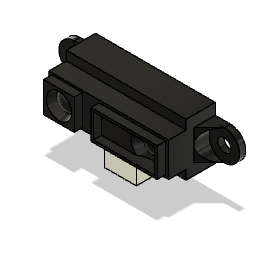
ApoioSensorIR v8 (Autodesk Fusion 360 archive; units mm, degrees)
design "GP2Y0A41SK0F"
Autodesk Fusion 360 part; units mm, degrees
sketch "Base" plane through (0, 0, 0) normal (0, 0, 1) x (1, 0, 0)
  line L0 (-14.75, 6.5) -> (14.75, 6.5)
  line L1 (14.75, 6.5) -> (14.75, -6.5)
  line L2 (14.75, -6.5) -> (-14.75, -6.5)
  line L3 (-14.75, -6.5) -> (-14.75, 6.5)
  line L4 (-18.5, 0) -> (18.5, 0) construction
  circle A0 centre (18.5, 0) radius 1.6
  circle A1 centre (18.5, 0) radius 3.75
  circle A2 centre (-18.5, 0) radius 1.6
  circle A3 centre (-18.5, 0) radius 3.75
  line L5 (-14.75, 3.75) -> (-18.5, 3.75)
  line L6 (14.75, 3.75) -> (18.5, 3.75)
  line L7 (-14.75, -3.75) -> (-18.5, -3.75)
  line L8 (14.75, -3.75) -> (18.5, -3.75)
  line L9 (-6.5, -3.75) -> (-14, -3.75)
  line L10 (-14, -3.75) -> (-14, 3.75)
  line L11 (-14, 3.75) -> (-6.5, 3.75)
  line L12 (-6.5, 3.75) -> (-6.5, -3.75)
  line L13 (-14.75, 4.2) -> (14.75, 4.2)
  line L14 (14.75, -4.2) -> (-14.75, -4.2)
  line L15 (-2.35, 3.6) -> (13.95, 3.6)
  line L16 (13.95, 3.6) -> (13.95, -3.6)
  line L17 (13.95, -3.6) -> (-2.35, -3.6)
  line L18 (-2.35, -3.6) -> (-2.35, 3.6)
  line L19 (-2.35, -3.6) -> (13.95, 3.6) construction
  line L20 (-14, -3.75) -> (-6.5, 3.75) construction
  line L21 (-14.75, -6.5) -> (14.75, 6.5) construction
  line L22 (13.35, -3) -> (-1.75, -3)
  line L23 (-1.75, -3) -> (-1.75, 3)
  line L24 (-1.75, 3) -> (13.35, 3)
  line L25 (13.35, 3) -> (13.35, -3)
  line L26 (0, 0) -> (0, -6.5) construction
  line L27 (-5.05, -6.5) -> (-5.05, -4.2)
  line L28 (5.05, -6.5) -> (5.05, -4.2)
  point P0 (-10.25, 0)
  point P1 (9.45, 0)
  point P2 (-10.25, 0)
  point P3 (5.8, 0)
  dimension "d1" = 29.5
  dimension "d2" = 13
  dimension "d3" = 37
  dimension "d4" = 3.2
  dimension "d5" = 7.5
  dimension "d6" = 19.7
  dimension "d7" = 4.5
  dimension "d8" = 7.5
  dimension "d9" = 7.5
  dimension "d10" = 8.4
  dimension "d11" = 4.2
  dimension "d12" = 16.3
  dimension "d13" = 7.2
  dimension "d14" = 4.15
  dimension "d16" = 0.6
  dimension "d62" = 10.1
  dimension "d63" = 5.05
  constraint horizontal L0
  constraint perpendicular L0 L1
  constraint parallel L0 L2
  constraint parallel L1 L3
  constraint coincident L26.start origin
  constraint perpendicular L1 L4
  constraint midpoint L26.start L4
  constraint coincident L4.end A0.centre
  constraint concentric A0 A1
  constraint coincident L4.start A2.centre
  constraint concentric A2 A3
  constraint equal A0 A2
  constraint equal A1 A3
  constraint coincident L3 L5.start
  constraint coincident A3 L5.end
  constraint parallel L0 L5
  constraint coincident L1 L6.start
  constraint coincident A1 L6.end
  constraint tangent A1 L6
  constraint parallel L0 L6
  constraint tangent A3 L5
  constraint coincident L3 L7.start
  constraint coincident A3 L7.end
  constraint tangent A3 L7
  constraint parallel L2 L7
  constraint coincident L1 L8.start
  constraint coincident A1 L8.end
  constraint tangent A1 L8
  constraint parallel L2 L8
  constraint coincident L4 P2
  constraint coincident L4 P1
  constraint horizontal L9
  constraint perpendicular L9 L10
  constraint parallel L9 L11
  constraint parallel L10 L12
  constraint coincident P2 P0
  constraint coincident L3 L13.start
  constraint coincident L1 L13.end
  constraint perpendicular L1 L13
  constraint coincident L1 L14.start
  constraint coincident L3 L14.end
  constraint perpendicular L3 L14
  constraint horizontal L15
  constraint perpendicular L15 L16
  constraint parallel L15 L17
  constraint parallel L16 L18
  constraint coincident L4 P3
  constraint midpoint P2 L20
  constraint midpoint P3 L19
  constraint midpoint L2 L26.end
  constraint perpendicular L2 L26
  constraint coincident L2 L27.start
  constraint coincident L14 L27.end
  constraint perpendicular L14 L27
  constraint coincident L2 L28.start
  constraint coincident L14 L28.end
  constraint perpendicular L14 L28
  measures "d1" distance of L1.end L2.end
  measures "d2" distance of L0.end L1.end
  measures "d3" distance of L4.start L4.end
  measures "d4" diameter of A0
  measures "d5" diameter of A1
  measures "d6" distance of P2 P1
  measures "d7" distance of L3 P2
  measures "d8" distance of L10.end L11.end
  measures "d9" distance of L9.end L10.end
  measures "d10" distance of L13 L14
  measures "d11" distance of L26.start L14
  measures "d12" distance of L16.end L17.end
  measures "d13" distance of L15.end L16.end
  measures "d14" distance of L12 L18
  measures "d62" distance of L27 L28
  measures "d63" distance of L26 L27
extrude "Extrude1" add sketch "Base" along normal blind 13.5 contours L9 L10 L11 L12 | L15 L16 L17 L18 makes body 1 at (-9, -3.75, 4.5) makes body 2 at (3.0833, 3.6, 4.5)
extrude "Extrude2" add sketch "Base" along normal blind 11.5 contours L1 L3 L13 L14 | L22 L23 L24 L25 bodies 1 2
extrude "Extrude3" add sketch "Base" along normal blind 7.2 contours L0 L1 L3 L13 | L2 L3 L14 L27 | L1 L2 L14 L28 bodies 1
extrude "Extrude10" add sketch "Base" along normal blind 3.3 contours L2 L14 L27 L28 bodies 1
sketch "Fixation" plane through (0, -6.5, 0) normal (0, -1, 0) x (1, 0, 0)
  line L0 (-14.75, 0) -> (14.75, 0)
  line L1 (14.75, 0) -> (14.75, 7.2)
  line L2 (14.75, 7.2) -> (5.05, 7.2)
  line L3 (-14.75, 7.2) -> (-14.75, 0)
  line L4 (14.75, 0) -> (18.5, 0)
  line L5 (14.75, 0) -> (14.75, 5.25)
  line L6 (18.5, 0) -> (18.5, 1.5)
  line L7 (14.75, 5.25) -> (18.5, 1.5)
  line L8 (0, 0) -> (0, 3) construction
  line L9 (-14.75, 5.25) -> (-18.5, 1.5)
  line L10 (-18.5, 0) -> (-18.5, 1.5)
  line L11 (-14.75, 0) -> (-18.5, 0)
  line L12 (-14.75, 0) -> (-14.75, 5.25)
  line L13 (5.05, 7.2) -> (5.05, 3.3)
  line L14 (-5.05, 3.3) -> (-5.05, 7.2)
  line L15 (5.05, 3.3) -> (-5.05, 3.3)
  line L16 (-5.05, 7.2) -> (-14.75, 7.2)
  dimension "d25" = 3.75
  dimension "d26" = 5.25
  dimension "d27" = 1.5
  constraint coincident L0.end L1.start
  constraint perpendicular L1 L4
  constraint perpendicular L0 L5
  constraint perpendicular L4 L6
  constraint coincident L8.start origin
  constraint perpendicular L0 L8
  constraint symmetric L0.end L8 L0.start
  constraint symmetric L4.end L8 L10.start
  constraint symmetric L5.end L8 L9.start
  constraint symmetric L6.end L8 L9.end
  measures "d25" distance of L0.end L4.end
  measures "d26" distance of L0.end L5.end
  measures "d27" distance of L4.end L6.end
extrude "Extrude5" add sketch "Fixation" along normal mid plane 7.5 from surface at -6.5 contours L3 L9 L10 L11 L12 | L1 L4 L5 L6 L7 bodies 1
extrude "Extrude6" cut sketch "Base" along normal through all contours A3 | A1 | A0 | A2 bodies 1
extrude "Extrude7" add sketch "Base" along normal blind 1.5 contours A3 | A1 bodies 1
ref_plane "WorkPlane2" through (5.8, 0, 10) normal (0, 0, 1) x (1, 0, 0)
sketch "Detector_Fitting1" plane through (0, 0, 11.5) normal (0, 0, 1) x (1, 0, 0)
  line L0 (13.35, 3) -> (-1.75, 3)
  line L1 (-1.75, 3) -> (-1.75, -3)
  line L2 (-1.75, -3) -> (13.35, -3)
  line L3 (13.35, -3) -> (13.35, 3)
  line L4 (0, 0) -> (9.45, 0) construction
  circle A0 centre (9.45, 0) radius 4
  dimension "d34" = 9.45
  dimension "d35" = 8
  constraint coincident L4.start origin
  constraint parallel L0 L4
  constraint coincident L4.end A0.centre
  measures "d34" distance of L4.start L4.end
  measures "d35" diameter of A0
sketch "Detector_Fitting2" plane through (5.8, 0, 10) normal (0, 0, 1) x (1, 0, 0)
  line L0 (0, 0) -> (3.625, 0)
  circle A0 centre (3.625, 0) radius 2.375
  dimension "d38" = 3.625
  dimension "d39" = 4.75
  constraint coincident L0.start origin
  constraint horizontal L0
  constraint coincident L0.end A0.centre
  measures "d38" distance of L0.start L0.end
  measures "d39" diameter of A0
loft "Loft1" cut profiles "Detector_Fitting1", "Detector_Fitting2" section 1 contours L0 L2 L3 A0 | L0 A0 | L3 A0 | L2 A0 section 2 bodies 1
extrude "Extrude8" add 1 faces at (-1.6833, -4.2, 10.0667) along direction (0, 1, 0) up to surface (1.2 mm away) on bodies 1 bodies 1
extrude "Extrude9" add 1 faces at (4.9167, 4.2, 10.0667) along direction (0, -1, 0) up to surface (1.2 mm away) on bodies 1 bodies 1
ref_plane "WorkPlane4" through (-10.25, 0, 11.5) normal (0, 0, 1) x (1, 0, 0)
sketch "Emitter_Fitting1" plane through (-10.25, 0, 11.5) normal (0, 0, 1) x (1, 0, 0)
  circle A0 centre (0, 0) radius 2.5
  dimension "d50" = 5
  constraint coincident A0.centre origin
  measures "d50" diameter of A0
sketch "Emitter_Fitting2" plane through (0, 0, 13.5) normal (0, 0, 1) x (1, 0, 0)
  line L0 (-6.5, 3.75) -> (-14, 3.75)
  line L1 (-14, 3.75) -> (-14, -3.75)
  line L2 (-14, -3.75) -> (-6.5, -3.75)
  line L3 (-6.5, -3.75) -> (-6.5, 3.75)
  line L4 (0, 0) -> (-10.25, 0) construction
  circle A0 centre (-10.25, 0) radius 3.125
  dimension "d51" = 10.25
  dimension "d52" = 6.25
  constraint coincident L4.start origin
  constraint horizontal L4
  constraint coincident L4.end A0.centre
  measures "d51" distance of L4.start L4.end
  measures "d52" diameter of A0
loft "Loft2" cut profiles "Emitter_Fitting2", "Emitter_Fitting1" section 1 contours A0 section 2 bodies 1
ref_plane "WorkPlane3" through (0, 0, 7.4) normal (0, -1, 0) x (1, 0, 0)
sketch "Emitter_Detector" plane through (0, 0, 0) normal (0, -1, 0) x (1, 0, 0)
  line L0 (-14.75, 7.2) -> (14.75, 7.2)
  line L1 (14.75, 7.2) -> (14.75, 11.5)
  line L2 (14.75, 11.5) -> (-14.75, 11.5)
  line L3 (-14.75, 11.5) -> (-14.75, 7.2)
  line L4 (9.45, 10) -> (9.45, 13.5577) construction
  line L5 (11.825, 10) -> (11.825, 13.5577) construction
  line L6 (7.075, 10) -> (7.075, 13.5577) construction
  circle A0 centre (9.45, 7.4291) radius 3.5
  line L7 (-14.75, 11.5) -> (-10.25, 11.5) construction
  line L8 (-10.25, 11.5) -> (-10.25, 14)
  line L9 (-7.75, 11.5) -> (-7.75, 14)
  line L10 (-12.75, 11.5) -> (-12.75, 14)
  line L11 (-10.25, 11.5) -> (-10.25, 5.5505)
  circle A1 centre (-10.25, 9.0505) radius 3.5
  line L12 (9.45, 10.9291) -> (9.45, 3.9291)
  point P0 (9.45, 10.9291)
  dimension "d45" = 2.375
  dimension "d46" = -2.375
  dimension "d47" = 7
  dimension "d53" = 4.5
  dimension "d54" = 2.5
  dimension "d55" = -2.5
  dimension "d56" = 7
  dimension "d59" = 1.5
  dimension "d60" = 5.3
  constraint coincident L5.start A0
  constraint perpendicular L3 L7
  constraint perpendicular L2 L8
  constraint perpendicular L2 L11
  constraint coincident L11 A1.centre
  constraint coincident L9.start A1
  constraint coincident L11.end A1
  constraint coincident L6.start A0
  constraint coincident L4 P0
  constraint coincident A0 P0
  constraint perpendicular L2 L4
  constraint coincident P0 L12.start
  constraint coincident A0 L12.end
  constraint parallel L4 L12
  measures "d47" diameter of A0
  measures "d53" distance of L2.end L7.end
  measures "d54" distance of L8
  measures "d55" distance of L8
  measures "d56" diameter of A1
  measures "d59" vertical distance of L1.end L5.start
  measures "d60" horizontal distance of L1.end A0.centre
revolve "Revolve1" add sketch "Emitter_Detector" angle 360 about axis through (9.45, 0, 10) along (0, 0, 1) separate body contours L0 A0 L12 | L0 A0 L12 picked at (9.2771, 9.6732) picked at (7.143, 7.0419) makes body 3
revolve "Revolve2" add sketch "Emitter_Detector" angle 360 about axis through (-10.25, 0, 11.5) along (0, 0, 1) separate body contours L0 L2 L11 A1 | L0 L11 A1 | L2 L8 A1 picked at (-9.1221, 9.5483) picked at (-10.0816, 6.1126) picked at (-10.0958, 12.1901) makes body 4
sketch "Connector_and_PCB" plane through (0, -4.2, 0) normal (0, -1, 0) x (1, 0, 0)
  line L0 (-5.05, 3.3) -> (5.05, 3.3)
  line L1 (5.05, 3.3) -> (5.05, 7.2)
  line L2 (5.05, 7.2) -> (14.75, 7.2)
  line L3 (14.75, 7.2) -> (14.75, 11.5)
  line L4 (14.75, 11.5) -> (-14.75, 11.5)
  line L5 (-14.75, 11.5) -> (-14.75, 7.2)
  line L6 (-14.75, 7.2) -> (-5.05, 7.2)
  line L7 (-5.05, 7.2) -> (-5.05, 3.3)
  line L8 (-5.05, 3.3) -> (5.05, 3.3)
  line L9 (5.05, 3.3) -> (5.05, 4.5)
  line L10 (5.05, 4.5) -> (-5.05, 4.5)
  line L11 (-5.05, 4.5) -> (-5.05, 3.3)
  line L12 (-3.9375, 4.5) -> (-3.9375, 8.625)
  line L13 (-3.9375, 8.625) -> (3.9375, 8.625)
  line L14 (3.9375, 8.625) -> (3.9375, 4.5)
  point P0 (0, 8.625)
  point P1 (0, 4.5)
  dimension "d66" = 10.1
  dimension "d67" = 1.2
  dimension "d68" = 4.125
  dimension "d69" = 7.875
  constraint coincident L0.start L7.end
  constraint perpendicular L7 L8
  constraint coincident L0.end L1.start
  constraint perpendicular L0 L9
  constraint coincident L7 L10.end
  constraint perpendicular L7 L10
  constraint coincident L10 L12.start
  constraint perpendicular L10 L12
  constraint perpendicular L12 L13
  constraint coincident L10 L14.end
  constraint perpendicular L10 L14
  constraint midpoint L13 P0
  constraint midpoint L10 P1
  constraint vertical P0 P1
  measures "d66" distance of L0.start L0.end
  measures "d67" distance of L0.end L9.end
  measures "d68" distance of L12.start L12.end
  measures "d69" distance of L12.end L13.end
extrude "Extrude11" add sketch "Connector_and_PCB" along normal blind 6.75 from surface at 1.45 separate body contours L10 L12 L13 L14 makes body 5
sketch "Connector_side" plane through (3.9375, 0, 0) normal (1, 0, 0) x (0, 0, -1)
  line L0 (-4.5, -5.65) -> (-8.625, -5.65)
  line L1 (-8.625, -5.65) -> (-8.625, -12.4)
  line L2 (-8.625, -12.4) -> (-4.5, -12.4)
  line L3 (-4.5, -12.4) -> (-4.5, -5.65)
  line L4 (-4.5, -12.4) -> (-4.5, -5.65)
  line L5 (-4.5, -12.4) -> (-8.625, -12.4)
  line L6 (-8.625, -12.4) -> (-8.625, -6.5)
  line L7 (-4.5, -5.65) -> (-7, -5.65)
  line L8 (-7, -5.65) -> (-8.625, -6.5)
  dimension "d73" = 5.9
  dimension "d75" = 2.5
  constraint coincident L2.end L3.start
  constraint coincident L0.start L3.end
  constraint coincident L1.end L2.start
  constraint perpendicular L2 L6
  constraint coincident L0 L7.end
  constraint perpendicular L3 L7
  measures "d73" distance of L1.end L6.end
  measures "d75" distance of L0.start L7.end
extrude "Extrude12" cut sketch "Connector_side" against normal up to surface (7.875 mm away) contours L0 L1 L2 L3 L4 L5 L6 L7 L8 keep common part bodies 5
shell "Shell1" thickness 0.3 removed faces 1 at (1.3125, -12.4, 5.875) on bodies 5
extrude "Extrude13" add sketch "Connector_and_PCB" along normal blind 8.2 separate body contours L0 L1 L7 L8 L9 L10 L11 makes body 6
equation "d26 = 3.75 mm + 1.5 mm"
equation "d45 = ( 4.75 / 2 ) * 1 mm"
equation "d46 = ( -4.75 / 2 ) * 1 mm"
named bodies: "Sensor", "Light_Detector", "Light_Emitter", "Connector", "PCB"
